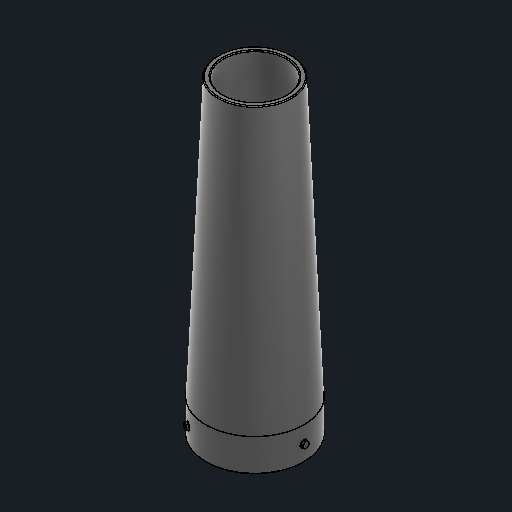
# Autodesk Inventor part: Tapered Vac Fitting
Saved by Autodesk Inventor 2026.2 (Build 302298000, 298)
## iProperties
Created: 2026-07-13
Part Number: Tapered Vac Fitting
Material: PVC, Unplasticized
Document SubType Name: Modeling
Designer: Joshua Eah
Density: 1.29 g/cm^3
Appearance: Smooth - Black
Author: Joshua Eah
Autodesk Inventor part; units mm, degrees
ref_plane "YZ Plane" through (0, 0, 0) normal (1, 0, 0) x (0, 1, 0)
ref_plane "XZ Plane" through (0, 0, 0) normal (0, 1, 0) x (-1, 0, 0)
ref_plane "XY Plane" through (0, 0, 0) normal (0, 0, 1) x (1, 0, 0)
sketch "Base Profile" plane through (0, 0, 0) normal (0, 1, 0) x (-1, 0, 0)
  circle A0 centre (0, 0) radius 22.45
  circle A1 centre (0, 0) radius 20
  dimension "d55" = 44.9
  dimension "d56" = 40
  constraints: 2 centre point, 2 coincident
  measures "d55" diameter of A0
  measures "d56" diameter of A1
extrude "Bayonet Mounting" add sketch "Base Profile" along normal blind 15
sketch "Profile" plane through (0, 0, 0) normal (0, 0, 1) x (1, 0, 0)
  line L0 (0, 0) -> (0, 15)
  line L1 (0, 15) -> (22.4, 15)
  line L2 (0, 0) -> (22.4, 0)
  line L3 (22.4, 15) -> (22.4, 0)
  line L4 (21.3, 9) -> (23.5, 9)
  line L5 (23.5, 9) -> (23.5, 6)
  line L6 (23.5, 6) -> (21.3, 6)
  line L7 (21.3, 6) -> (21.3, 9)
  line L8 (21.3, 9) -> (23.5, 6) construction
  line L9 (23.5, 9) -> (21.3, 6) construction
  line L10 (23.5, 7.5) -> (21.3, 7.5)
  line L11 (22.4, 15) -> (16.8551, 142)
  line L12 (16.8551, 142) -> (0, 142)
  line L13 (0, 142) -> (0, 15)
  line L14 (14.4551, 142) -> (20, 15)
  point P0 (22.4, 7.5)
  dimension "d59" = 15
  dimension "d60" = 44.8
  dimension "d106" = 1.1
  dimension "d107" = 3
  dimension "d113" = 127
  dimension "d114" = 87.5
  dimension "d117" = 40
  constraints: 30 end point, 5 midpoint, 4 horizontal, 3 parallel, 2 point on line, 2 vertical, 1 coincident, 1 collinear, 1 perpendicular
  measures "d59" distance of L0.start L0.end
  measures "d60" diameter of L3 L0
  measures "d106" distance between parallel lines of L5 L3
  measures "d107" distance of L4.end L5.end
  measures "d113" distance from line of L1 L11.end
  measures "d114" angle of L1 L11
  measures "d117" diameter of L14.end L0
revolve "Lug" add sketch "Profile" angle 360 about axis through (23.5, 7.5, 0) along (-1, 0, 0) contours L10 L7 L4 L3 | L3 L4 L5 L10
chamfer "Lug Chamfer" distance 0.2 angle 45 2 edges at (22.45, 6, 0.0029) (23.5, 6, 0)
pattern_circular "Lugs" count 3 over 360 about axis through (0, -10, 0) along (0, 1, 0) of "Lug", "Lug Chamfer"
revolve "Top Section" add sketch "Profile" angle 360 about axis through (0, 142, 0) along (0, -1, 0) contours L14 L12 L11 L1
fillet "Bottom Edge Fillets" radius 0.4 4 edges at (22.45, 0, 0) (20, 0, 0) (-14.4551, 142, 0) (-16.8551, 142, 0)
equation "\"lugThickness\" = 1.3"
equation "\"lugHeight\" = 3"
body "Solid2"
